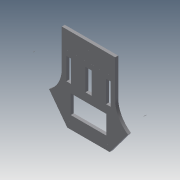
# Autodesk Inventor part: zak.-deska_ruka_(sablona)
Saved by Autodesk Inventor 2013 (Build 170138000, 138)
## iProperties
Created: 2013-02-01
Part Number: zak.-deska_ruka_(sablona)
Material: Generic
Document SubType Name: Modeling
Designer: idle-rug
Density: 1 g/cm^3
Author: idle-rug
Autodesk Inventor part; units mm, degrees
(part 1 of 2)
ref_plane "YZ Plane" through (0, 0, 0) normal (1, 0, 0) x (0, 1, 0)
ref_plane "XZ Plane" through (0, 0, 0) normal (0, 1, 0) x (-1, 0, 0)
ref_plane "XY Plane" through (0, 0, 0) normal (0, 0, 1) x (1, 0, 0)
sketch "Sketch1" plane through (0, 0, 0) normal (0, 1, 0) x (-1, 0, 0)
  line L0 (0, -20) -> (10, -20)
  line L1 (10, -20) -> (25, 0)
  line L2 (0, -20) -> (-10, -20)
  line L3 (-10, -20) -> (-25, 0)
  line L4 (25, 0) -> (25, 10)
  line L5 (0, 20) -> (15, 20)
  line L6 (15, 20) -> (25, 10)
  line L7 (0, 20) -> (-15, 20)
  line L8 (-25, 0) -> (-25, 10)
  line L9 (-25, 10) -> (-15, 20)
  line L10 (0, 20) -> (0, -20)
  point P0 (0, 0)
  dimension "d2" = 10
  dimension "d3" = 10
  dimension "d4" = 10
  dimension "d7" = 10
  constraints: 22 end point, 1 parallel
  measures "d2" distance of L0.start L0.end
  measures "d3" distance of L0.start L2.end
  measures "d4" distance of L1.end L4.end
  measures "d7" distance of L3.end L8.end
extrude "Extrusion1" add sketch "Sketch1" along normal blind 2
sketch "Sketch2" plane through (0, 2, 0) normal (0, 1, 0) x (1, 0, 0)
  circle A0 centre (-10, 10) radius 1.5
  circle A1 centre (10, 10) radius 1.5
  circle A2 centre (-16, 2) radius 1.5
  circle A3 centre (16, 2) radius 1.5
  point P0 (0, 0)
  dimension "d11" = 3
  dimension "d12" = 3
  dimension "d14" = 3
  dimension "d15" = 3
  constraints: 4 centre point
  measures "d11" diameter of A0
  measures "d12" diameter of A1
  measures "d14" diameter of A2
  measures "d15" diameter of A3
extrude "Extrusion2" cut sketch "Sketch2" against normal blind 10
sketch "Sketch4" plane through (0, 2, 0) normal (0, 1, 0) x (1, 0, 0)
  line L0 (25, -10) -> (25, 0) projected
  line L1 (-10, 20) -> (-10, 14)
  circle A0 centre (-10, 14) radius 1.5
  line L2 (10, 20) -> (10, 14)
  circle A1 centre (10, 14) radius 1.5
  point P0 (0, 0)
  dimension "d20" = 6
  dimension "d21" = 3
  dimension "d22" = 6
  dimension "d23" = 3
  constraints: 4 end point, 2 centre point, 2 coincident, 2 parallel
  measures "d20" distance of L1.start L1.end
  measures "d21" diameter of A0
  measures "d22" distance of L2.start L2.end
  measures "d23" diameter of A1
extrude "Extrusion3" cut sketch "Sketch4" against normal blind 10
sketch "Sketch5" plane through (0, 2, 0) normal (0, 1, 0) x (1, 0, 0)
  circle A0 centre (-10, 10) radius 1.5 projected
  circle A1 centre (10, 10) radius 1.5 projected
extrude "Extrusion4" add sketch "Sketch5" against normal blind 2
sketch "Sketch6" plane through (0, 2, 0) normal (0, 1, 0) x (1, 0, 0)
  circle A0 centre (-19, 2) radius 1.5
  circle A1 centre (19, 2) radius 1.5
  dimension "d34" = 3
  dimension "d36" = 3
  constraints: 2 centre point
  measures "d34" diameter of A0
  measures "d36" diameter of A1
extrude "Extrusion5" cut sketch "Sketch6" against normal blind 2
sketch "Sketch7" plane through (0, 2, 0) normal (0, 1, 0) x (1, 0, 0)
  circle A0 centre (-16, 2) radius 1.5 projected
  circle A1 centre (16, 2) radius 1.5 projected
  point P0 (-17.5, 2)
  point P1 (17.5, 2)
  point P2 (0, 0)
  constraints: 2 horizontal alignment
extrude "Extrusion6" add sketch "Sketch7" against normal blind 2
sketch "Sketch9" plane through (0, 2, 0) normal (0, 1, 0) x (1, 0, 0)
  line L0 (0, -2) -> (0, -4)
  circle A0 centre (0, -4) radius 2
  line L1 (-2, -4) -> (-2, -16)
  line L2 (-2, -16) -> (2, -16)
  line L3 (2, -4) -> (2, -16)
  circle A1 centre (0, -16) radius 2
  point P0 (0, 0)
  dimension "d48" = 2
  dimension "d49" = 4
  dimension "d51" = 12
  dimension "d52" = 4
  constraints: 8 end point, 2 centre point, 2 point on circle, 1 coincident, 1 midpoint, 1 perpendicular, 1 tangent
  measures "d48" distance of L0.start L0.end
  measures "d49" diameter of A0
  measures "d51" distance of L1.start L1.end
  measures "d52" diameter of A1
extrude "Extrusion7" cut sketch "Sketch9" against normal blind 2
sketch "Sketch10" plane through (0, 2, 0) normal (0, 1, 0) x (1, 0, 0)
  line L0 (-2, -16) -> (-2, -4) projected
  arc A0 (2, -4) -> (-2, -4) centre (0, -4) ccw projected
  line L1 (2, -4) -> (2, -16) projected
  arc A1 (-2, -16) -> (2, -16) centre (0, -16) ccw projected
  line L2 (25, -10) -> (25, 0) projected
  line L3 (0, -2) -> (0, -3.8)
  line L4 (0, -3.8) -> (0, -5.8)
  circle A2 centre (0, -5.8) radius 2
  point P0 (0, 0)
  dimension "d55" = 1.8
  dimension "d56" = 2
  dimension "d57" = 4
  constraints: 4 end point, 1 centre point, 1 coincident, 1 parallel, 1 point on circle, 1 point on line
  measures "d55" distance of L3.start L3.end
  measures "d56" distance of L3.end L4.end
  measures "d57" diameter of A2
extrude "Extrusion8" add sketch "Sketch10" against normal blind 2 contours L0 A2 L1 A1 | L0 A0 L3 A2 | L3 A0 L1 A2
sketch "Sketch11" plane through (0, 2, 0) normal (0, 1, 0) x (1, 0, 0)
  circle A0 centre (0, -5.8) radius 2 projected
  line L0 (25, -10) -> (25, 0) projected
  line L1 (2, -5.8) -> (2, -17.8)
  line L2 (2, -17.8) -> (-2, -17.8)
  line L3 (-2, -17.8) -> (-2, -5.8)
  circle A1 centre (0, -17.8) radius 2
  point P0 (0, 0)
  dimension "d60" = 12
  dimension "d61" = 4
  dimension "d62" = 4
  constraints: 6 end point, 2 point on circle, 2 tangent, 1 centre point, 1 midpoint, 1 parallel, 1 perpendicular
  measures "d60" distance of L1.start L1.end
  measures "d61" distance of L1.end L2.end
  measures "d62" diameter of A1
extrude "Extrusion9" cut sketch "Sketch11" against normal blind 2
sketch "Sketch12" plane through (0, 2, 0) normal (0, 1, 0) x (1, 0, 0)
  line L0 (-2, -17.8) -> (-2, -5.8) projected
  arc A0 (2, -5.8) -> (-2, -5.8) centre (0, -5.8) ccw projected
  line L1 (2, -5.8) -> (2, -17.8) projected
  arc A1 (-2, -17.8) -> (2, -17.8) centre (0, -17.8) ccw projected
  line L2 (-2, -5.8) -> (-2, -16.2)
  line L3 (-2, -16.2) -> (2, -16.2)
  line L4 (2, -16.2) -> (2, -5.8)
  line L5 (-2, -5.8) -> (2, -5.8)
  point P0 (0, 0)
  dimension "d65" = 16
  dimension "d66" = 12
  dimension "d67" = 10.4
  constraints: 8 end point, 2 perpendicular, 2 point on line, 1 collinear, 1 tangent
  measures "d66" distance of A1.centre A0.centre
  measures "d67" distance of L0.end L2.end
extrude "Extrusion10" add sketch "Sketch12" against normal blind 2 contours L0 L3 L1 A1
sketch "Sketch13" plane through (0, 2, 0) normal (0, 1, 0) x (1, 0, 0)
  line L0 (2, -16.2) -> (-2, -16.2) projected
  circle A0 centre (0, -16.2) radius 2
  point P0 (0, 0)
  dimension "d70" = 4
  constraints: 1 centre point, 1 midpoint
  measures "d70" diameter of A0
extrude "Extrusion11" cut sketch "Sketch13" against normal blind 2
sketch "Sketch14" plane through (0, 0, 0) normal (0, -1, 0) x (1, 0, 0)
  line L0 (15, 20) -> (25, 10) projected
  line L1 (-15, 20) -> (15, 20) projected
  line L2 (-25, 10) -> (-15, 20) projected
  line L3 (-25, 0) -> (-25, 10) projected
  line L4 (-15, 20) -> (-15, 40)
  line L5 (-15, 40) -> (15, 40)
  line L6 (15, 40) -> (15, 20)
  line L7 (15, 40) -> (25, 10)
  line L8 (-25, 10) -> (-15, 40)
  point P0 (0, 0)
  dimension "d74" = 20
  dimension "d75" = 30
  constraints: 10 end point, 1 parallel, 1 perpendicular
  measures "d74" distance of L1.start L4.end
  measures "d75" distance of L4.end L5.end
extrude "Extrusion12" add sketch "Sketch14" against normal blind 2
sketch "Sketch15" plane through (0, 2, 0) normal (0, 1, 0) x (1, 0, 0)
  circle A0 centre (-13.95, -27.8) radius 1.15
  circle A1 centre (13.95, -27.8) radius 1.15
  point P0 (0, 0)
  dimension "d83" = 2.3
  dimension "d84" = 2.3
  constraints: 2 centre point
  measures "d83" diameter of A0
  measures "d84" diameter of A1
extrude "Extrusion13" cut sketch "Sketch15" against normal blind 2
sketch "Sketch17" plane through (0, 0, 0) normal (0, -1, 0) x (1, 0, 0)
  line L0 (25, 10) -> (25, 0) projected
  line L1 (-25, 0) -> (-25, 10) projected
  arc A0 (-23.2, -2.4) -> (-19.7434, 25.7698) centre (-40.683, 14.0422) ccw
  arc A1 (19.7434, 25.7698) -> (23.2, -2.4) centre (40.683, 14.0422) ccw
  line L2 (-25, 0) -> (-23.2, -2.4)
  line L3 (19.7434, 25.7698) -> (25, 10)
  line L4 (25, 10) -> (25, 0)
  line L5 (23.2, -2.4) -> (25, 0)
  line L6 (-19.7434, 25.7698) -> (-25, 10)
  line L7 (-25, 0) -> (-25, 10)
  dimension "d90" = 24
  dimension "d92" = 24
  constraints: 12 end point, 4 point on circle, 2 centre point, 2 collinear
  measures "d90" radius of A0
  measures "d92" radius of A1
extrude "Extrusion14" cut sketch "Sketch17" against normal blind 2
sketch "Sketch18" plane through (0, 0, 0) normal (0, -1, 0) x (1, 0, 0)
  circle A0 centre (-11.2167, 36) radius 1.5
  circle A1 centre (11.2167, 36) radius 1.5
  circle A2 centre (0, -6.2) radius 1.5
  point P0 (0, 0)
  dimension "d97" = 3
  dimension "d98" = 3
  dimension "d100" = 3
  constraints: 3 centre point
  measures "d97" diameter of A0
  measures "d98" diameter of A1
  measures "d100" diameter of A2
extrude "Extrusion15" cut sketch "Sketch18" against normal blind 2
sketch "Sketch19" plane through (0, 0, 0) normal (0, -1, 0) x (1, 0, 0)
  circle A0 centre (11.2167, 36) radius 1.5 projected
  circle A1 centre (-11.2167, 36) radius 1.5 projected
  point P0 (0, 0)
extrude "Extrusion16" add sketch "Sketch19" against normal blind 2
sketch "Sketch20" plane through (0, 0, 0) normal (0, -1, 0) x (1, 0, 0)
  line L0 (19.7434, 25.7698) -> (15, 40) projected
  line L1 (-15, 40) -> (-19.7434, 25.7698) projected
  line L2 (10, -20) -> (-10, -20) projected
  line L3 (-19.7434, 25.7698) -> (-19.7434, 40)
  line L4 (-19.7434, 40) -> (19.7434, 40)
  line L5 (19.7434, 40) -> (19.7434, 25.7698)
  line L6 (-15, 40) -> (-19.7434, 25.7698)
  line L7 (19.7434, 25.7698) -> (15, 40)
  line L8 (-19.7434, 40) -> (-15, 40)
  line L9 (15, 40) -> (19.7434, 40)
  point P0 (0, 0)
  constraints: 14 end point, 3 collinear, 3 perpendicular
extrude "Extrusion17" add sketch "Sketch20" against normal blind 2
sketch "Sketch22" plane through (0, 0, 0) normal (0, -1, 0) x (1, 0, 0)
  circle A0 centre (0, -6.2) radius 1.5 projected
  circle A1 centre (19, -2) radius 1.5 projected
  circle A2 centre (-19, -2) radius 1.5 projected
  circle A3 centre (10, -14) radius 1.5 projected
  circle A4 centre (-10, -14) radius 1.5 projected
  circle A5 centre (13.95, 27.8) radius 1.15 projected
  circle A6 centre (-13.95, 27.8) radius 1.15 projected
  line L0 (19.7434, 25.7698) -> (19.7434, 40) projected
  line L1 (19.7434, 40) -> (-19.7434, 40) projected
  line L2 (-19.7434, 40) -> (-15.7434, 40)
  line L3 (-15.7434, 40) -> (-15.7434, 36)
  circle A7 centre (-15.7434, 36) radius 1.5
  circle A8 centre (-13.95, 27.8) radius 1.5
  circle A9 centre (-19, -2) radius 1.5
  circle A10 centre (0, -6.2) radius 1.5
  circle A11 centre (19, -2) radius 1.5
  circle A12 centre (-10, -14) radius 1.5
  circle A13 centre (10, -14) radius 1.5
  line L4 (19.7434, 36) -> (15.7434, 36)
  circle A14 centre (15.7434, 36) radius 1.5
  circle A15 centre (13.95, 27.8) radius 1.5
  circle A16 centre (15.7434, 36) radius 1.5
  point P0 (0, 0)
  dimension "d111" = 4
  dimension "d112" = 4
  dimension "d113" = 3
  dimension "d114" = 3
  dimension "d116" = 3
  dimension "d117" = 3
  dimension "d118" = 3
  dimension "d119" = 3
  dimension "d120" = 3
  dimension "d121" = 4
  dimension "d122" = 3
  dimension "d123" = 3
  dimension "d124" = 3
  constraints: 10 centre point, 10 coincident, 6 end point, 2 perpendicular, 2 point on line
  measures "d111" distance of L1.end L2.end
  measures "d112" distance of L2.end L3.end
  measures "d113" diameter of A7
  measures "d114" diameter of A8
  measures "d116" diameter of A9
  measures "d117" diameter of A10
  measures "d118" diameter of A11
  measures "d119" diameter of A12
  measures "d120" diameter of A13
  measures "d121" distance of L4.start L4.end
  measures "d122" diameter of A14
  measures "d123" diameter of A15
  measures "d124" diameter of A16
extrude "Extrusion18" cut sketch "Sketch22" against normal blind 2 contours A7 | A8 | A14 | A15
sketch "Sketch23" plane through (0, 0, 0) normal (0, -1, 0) x (1, 0, 0)
  circle A0 centre (-13.95, 27.8) radius 1.5 projected
  circle A1 centre (13.95, 27.8) radius 1.5 projected
  circle A2 centre (-13.95, 27.8) radius 1.15
  circle A3 centre (13.95, 27.8) radius 1.15
  circle A4 centre (10, 16.2) radius 2
  circle A5 centre (10, 5.8) radius 2
  line L0 (8, 16.2) -> (8, 5.8)
  line L1 (12, 16.2) -> (12, 5.8)
  line L2 (8, 5.8) -> (12, 5.8)
  line L3 (8, 16.2) -> (12, 16.2)
  point P0 (0, 0)
  dimension "d131" = 4
  dimension "d127" = 2.3
  dimension "d128" = 2.3
  dimension "d132" = 4
  constraints: 8 end point, 4 point on circle, 3 centre point, 2 coincident, 2 parallel, 2 vertical, 1 horizontal alignment, 1 perpendicular, 2 other
  measures "d127" diameter of A2
  measures "d128" diameter of A3
  measures "d132" diameter of A5
extrude "Extrusion19" cut sketch "Sketch23" against normal blind 2
sketch "Sketch24" plane through (0, 0, 0) normal (0, -1, 0) x (1, 0, 0)
  circle A0 centre (-13.95, 27.8) radius 1.5 projected
  circle A1 centre (13.95, 27.8) radius 1.5 projected
  circle A2 centre (-13.95, 27.8) radius 1.15
  circle A3 centre (13.95, 27.8) radius 1.15
  point P0 (0, 0)
  dimension "d135" = 2.3
  dimension "d136" = 2.3
  constraints: 2 centre point, 2 coincident
  measures "d135" diameter of A2
  measures "d136" diameter of A3
extrude "Extrusion20" add sketch "Sketch24" against normal blind 2
sketch "Sketch25" plane through (0, 0, 0) normal (0, -1, 0) x (1, 0, 0)
  circle A0 centre (0, -14) radius 1.5
  point P0 (0, 0)
  dimension "d139" = 3
  constraints: 1 centre point
  measures "d139" diameter of A0
extrude "Extrusion21" cut sketch "Sketch25" against normal blind 2
sketch "Sketch26" plane through (0, 0, 0) normal (0, -1, 0) x (1, 0, 0)
  circle A0 centre (0, -6.2) radius 1.5 projected
  point P0 (0, 0)
extrude "Extrusion22" add sketch "Sketch26" against normal blind 2
sketch "Sketch27" plane through (0, 0, 0) normal (0, -1, 0) x (1, 0, 0)
  arc A0 (19.7434, 25.7698) -> (23.2, -2.4) centre (40.683, 14.0422) ccw projected
  line L0 (19.7434, 25.7698) -> (19.7434, 40) projected
  line L1 (-19.7434, 40) -> (-19.7434, 25.7698) projected
  arc A1 (-23.2, -2.4) -> (-19.7434, 25.7698) centre (-40.683, 14.0422) ccw projected
  line L2 (0, 40) -> (-20, 40)
  line L3 (-20, 40) -> (-20, 26)
  line L4 (0, 40) -> (20, 40)
  line L5 (20, 40) -> (20, 26)
  arc A2 (-23.2, -2.4) -> (-20, 26) centre (-40.7609, 13.959) ccw
  arc A3 (20, 26) -> (23.2, -2.4) centre (40.7609, 13.959) ccw
  arc A4 (-23.2, -2.4) -> (-19.7434, 25.7698) centre (-40.683, 14.0422) ccw
  line L6 (-19.7434, 40) -> (-19.7434, 25.7698)
  line L7 (-20, 40) -> (-19.7434, 40)
  line L8 (19.7434, 40) -> (20, 40)
  line L9 (20, 40) -> (20, 26)
  line L10 (19.7434, 40) -> (19.7434, 25.7698)
  arc A5 (19.7434, 25.7698) -> (23.2, -2.4) centre (40.683, 14.0422) ccw
  point P0 (0, 0)
  dimension "d144" = 20
  dimension "d145" = 14
  dimension "d146" = 20
  dimension "d147" = 24
  dimension "d148" = 24
  constraints: 18 end point, 8 point on circle, 4 centre point, 3 collinear, 3 concentric, 3 perpendicular
  measures "d144" distance of L2.start L2.end
  measures "d145" distance of L2.end L3.end
  measures "d146" distance of L2.start L4.end
  measures "d147" radius of A2
  measures "d148" radius of A3
extrude "Extrusion23" add sketch "Sketch27" against normal blind 2
sketch "Sketch28" plane through (0, 0, 0) normal (0, -1, 0) x (1, 0, 0)
  circle A0 centre (15.7434, 36) radius 1.5 projected
  circle A1 centre (-15.7434, 36) radius 1.5 projected
  point P0 (0, 0)
extrude "Extrusion24" add sketch "Sketch28" against normal blind 2
sketch "Sketch29" plane through (0, 0, 0) normal (0, -1, 0) x (1, 0, 0)
  line L0 (20, 40) -> (16, 40)
  line L1 (20, 36) -> (20, 40)
  line L2 (-20, 40) -> (-16, 40)
  line L3 (-20, 36) -> (-20, 40)
  circle A0 centre (-16, 36) radius 1.5
  circle A1 centre (16, 36) radius 1.5
  point P0 (0, 0)
  dimension "d157" = 3
  dimension "d158" = 3
  constraints: 8 end point, 2 centre point, 2 horizontal
  measures "d157" diameter of A0
  measures "d158" diameter of A1
extrude "Extrusion25" cut sketch "Sketch29" against normal blind 2
sketch "Sketch30" plane through (0, 0, 0) normal (0, -1, 0) x (1, 0, 0)
  arc A0 (20, 26) -> (23.2, -2.4) centre (40.7609, 13.959) ccw projected
  arc A1 (-23.2, -2.4) -> (-20, 26) centre (-40.7609, 13.959) ccw projected
  arc A2 (20, 26) -> (23.2, -2.4) centre (35.5049, 13.3667) ccw
  arc A3 (-23.2, -2.4) -> (-20, 26) centre (-35.5049, 13.3667) ccw
  arc A4 (-23.2, -2.4) -> (-20, 26) centre (-40.7609, 13.959) ccw
  arc A5 (20, 26) -> (23.2, -2.4) centre (40.7609, 13.959) ccw
  point P0 (0, 0)
  dimension "d161" = 20
  dimension "d162" = 20
  constraints: 9 point on circle, 4 centre point, 2 concentric
  measures "d161" radius of A2
  measures "d162" radius of A3
extrude "Extrusion26" cut sketch "Sketch30" against normal blind 2
sketch "Sketch31" plane through (0, 0, 0) normal (0, -1, 0) x (1, 0, 0)
  circle A0 centre (-16, 36) radius 1.5 projected
  circle A1 centre (16, 36) radius 1.5 projected
  point P0 (0, 0)
extrude "Extrusion27" add sketch "Sketch31" against normal blind 2
sketch "Sketch32" plane through (0, 0, 0) normal (0, -1, 0) x (1, 0, 0)
  line L0 (-20, 40) -> (-17, 40)
  line L1 (-17, 40) -> (-17, 37)
  line L2 (-17, 37) -> (-20, 37)
  line L3 (-20, 37) -> (-20, 40)
  line L4 (20, 40) -> (17, 40)
  line L5 (17, 40) -> (17, 37)
  line L6 (17, 37) -> (20, 37)
  line L7 (20, 37) -> (20, 40)
  circle A0 centre (17, 37) radius 1.25
  circle A1 centre (-17, 37) radius 1.25
  point P0 (0, 0)
  dimension "d167" = 3
  dimension "d168" = 3
  dimension "d169" = 3
  dimension "d170" = 3
  dimension "d171" = 2.5
  dimension "d172" = 2.5
  constraints: 16 end point, 4 parallel, 2 centre point, 2 coincident, 2 horizontal, 2 perpendicular
  measures "d167" distance of L1.end L2.end
  measures "d168" distance of L0.end L1.end
  measures "d169" distance of L6.end L5.end
  measures "d170" distance of L5.end L4.end
  measures "d171" diameter of A0
  measures "d172" diameter of A1
extrude "Extrusion28" cut sketch "Sketch32" against normal blind 2 contours A1 L2 L1 | L1 L2 A1 | A0 L6 L5 | L5 L6 A0
sketch "Sketch33" plane through (-20, 0, 40) normal (0, 0, 1) x (1, 0, 0)
  line L0 (40, 0) -> (0, 0) projected
  line L1 (40, 0) -> (40, 2) projected
  line L2 (0, 2) -> (40, 2) projected
  line L3 (0, 0) -> (0, 2) projected
  point P0 (20, 0)
extrude "Extrusion29" add sketch "Sketch33" along normal blind 2
sketch "Sketch34" plane through (0, 2, 0) normal (0, 1, 0) x (1, 0, 0)
  arc A0 (23.2, 2.4) -> (20, -26) centre (35.5049, -13.3667) ccw projected
  line L0 (23.2, 2.4) -> (10, 20) projected
  line L1 (10, 20) -> (-10, 20) projected
  line L2 (-10, 20) -> (-23.2, 2.4) projected
  arc A1 (-20, -26) -> (-23.2, 2.4) centre (-35.5049, -13.3667) ccw projected
  line L3 (-20, -26) -> (-20, -42) projected
  line L4 (20, -42) -> (-20, -42) projected
  line L5 (20, -26) -> (20, -42) projected
  line L6 (0, 20) -> (-12.5, 20)
  line L7 (0, 20) -> (12.5, 20)
  line L8 (20, -42) -> (22.5, -42)
  line L9 (-20, -42) -> (-22.5, -42)
  line L10 (-22.5, -42) -> (-22.5, -26)
  line L11 (22.5, -42) -> (22.5, -26)
  line L12 (-12.5, 20) -> (-24.5, 4)
  line L13 (12.5, 20) -> (24.5, 4)
  arc A2 (-22.5, -26) -> (-24.5, 4) centre (-43.4307, -12.3287) ccw
  arc A3 (24.5, 4) -> (22.5, -26) centre (43.4307, -12.3287) ccw
  line L14 (20, -42) -> (20, -26)
  line L15 (-10, 20) -> (-23.2, 2.4)
  line L16 (10, 20) -> (23.2, 2.4)
  arc A4 (23.2, 2.4) -> (20, -26) centre (35.5049, -13.3667) ccw
  arc A5 (-20, -26) -> (-23.2, 2.4) centre (-35.5049, -13.3667) ccw
  line L17 (-20, -42) -> (-20, -26)
  point P0 (0, 0)
  dimension "d178" = 12.5
  dimension "d179" = 12.5
  dimension "d180" = 2.5
  dimension "d181" = 2.5
  dimension "d183" = 20
  dimension "d185" = 20
  dimension "d186" = 25
  dimension "d187" = 25
  constraints: 24 end point, 9 point on circle, 5 collinear, 4 centre point, 4 parallel, 2 concentric, 2 point on line, 1 midpoint, 1 perpendicular
  measures "d178" distance of L6.start L6.end
  measures "d179" distance of L6.start L7.end
  measures "d180" distance of L4.start L8.end
  measures "d181" distance of L3.end L9.end
  measures "d183" distance of L6.end L12.end
  measures "d185" distance of L7.end L13.end
  measures "d186" radius of A2
  measures "d187" radius of A3
extrude "Extrusion30" add sketch "Sketch34" against normal blind 2 contours L0 L7 L13 A3 L11 L8 L5 A0 | L9 L10 A2 L12 L6 L2 A1 L3
sketch "Sketch35" plane through (0, 2, 0) normal (0, 1, 0) x (1, 0, 0)
  line L0 (-12.5, 20) -> (-24.5, 4) projected
  arc A0 (-22.5, -26) -> (-24.5, 4) centre (-43.4307, -12.3287) ccw projected
  line L1 (22.5, -42) -> (22.5, -26) projected
  arc A1 (24.5, 4) -> (22.5, -26) centre (43.4307, -12.3287) ccw projected
  line L2 (24.5, 4) -> (12.5, 20) projected
  line L3 (-22.5, -42) -> (-24, -42)
  line L4 (-24, -42) -> (-24, -26)
  line L5 (22.5, -42) -> (24, -42)
  line L6 (24, -42) -> (24, -26)
  line L7 (12.5, 20) -> (14, 20)
  line L8 (14, 20) -> (26, 4)
  line L9 (-12.5, 20) -> (-14, 20)
  line L10 (-14, 20) -> (-26, 4)
  arc A2 (-24, -26) -> (-26, 4) centre (-43.6669, -12.2445) ccw
  arc A3 (26, 4) -> (24, -26) centre (43.6669, -12.2445) ccw
  line L11 (22.5, -42) -> (22.5, -26)
  line L12 (-22.5, -42) -> (-22.5, -26)
  line L13 (-24.5, 4) -> (-12.8, 19.6)
  line L14 (12.5, 20) -> (24.5, 4)
  arc A4 (-22.5, -26) -> (-24.5, 4) centre (-43.4307, -12.3287) ccw
  arc A5 (24.5, 4) -> (22.5, -26) centre (43.4307, -12.3287) ccw
  point P0 (0, 0)
  dimension "d190" = 1.5
  dimension "d191" = 1.5
  dimension "d192" = 1.5
  dimension "d193" = 20
  dimension "d194" = 1.5
  dimension "d195" = 20
  dimension "d196" = 24
  dimension "d197" = 24
  constraints: 24 end point, 8 point on circle, 7 equal length, 4 centre point, 4 perpendicular, 3 concentric, 1 point on line
  measures "d190" distance of L3.start L3.end
  measures "d191" distance of L1.start L5.end
  measures "d192" distance of L2.end L7.end
  measures "d193" distance of L7.end L8.end
  measures "d194" distance of L0.start L9.end
  measures "d195" distance of L9.end L10.end
  measures "d196" radius of A2
  measures "d197" radius of A3
extrude "Extrusion31" add sketch "Sketch35" against normal blind 2
sketch "Sketch36" plane through (0, 2, 0) normal (0, 1, 0) x (1, 0, 0)
  circle A0 centre (19, 2) radius 1.5 projected
  circle A1 centre (-19, 2) radius 1.5 projected
  circle A2 centre (10, 14) radius 1.5 projected
  circle A3 centre (-10, 14) radius 1.5 projected
  line L0 (-14, 20) -> (-26, 4) projected
  line L1 (26, 4) -> (14, 20) projected
  line L2 (10, 14) -> (19, 2)
  line L3 (-19, 2) -> (-10, 14)
  line L4 (-10, 14) -> (-12.72, 16.04)
  line L5 (-19, 2) -> (-21.72, 4.04)
  line L6 (10, 14) -> (12.72, 16.04)
  line L7 (12.72, 16.04) -> (21.72, 4.04)
  circle A4 centre (-21.72, 4.04) radius 1.5
  circle A5 centre (-12.72, 16.04) radius 1.5
  circle A6 centre (12.72, 16.04) radius 1.5
  circle A7 centre (21.72, 4.04) radius 1.5
  point P0 (0, 0)
  dimension "d200" = 3.4
  dimension "d201" = 3.4
  dimension "d202" = 3
  dimension "d203" = 3
  dimension "d204" = 3
  dimension "d205" = 3
  constraints: 12 end point, 4 centre point, 4 coincident, 4 parallel, 2 perpendicular
  measures "d200" distance of L3.end L4.end
  measures "d201" distance of L2.start L6.end
  measures "d202" diameter of A4
  measures "d203" diameter of A5
  measures "d204" diameter of A6
  measures "d205" diameter of A7
extrude "Extrusion32" cut sketch "Sketch36" against normal blind 2 contours A6 L7 L6 | L6 L7 A6 | A4 | A5 | A7
sketch "Sketch37" plane through (0, 2, 0) normal (0, 1, 0) x (1, 0, 0)
  circle A0 centre (19, 2) radius 1.5 projected
  circle A1 centre (-19, 2) radius 1.5 projected
  circle A2 centre (10, 14) radius 1.5 projected
  circle A3 centre (-10, 14) radius 1.5 projected
  point P0 (0, 0)
extrude "Extrusion33" add sketch "Sketch37" against normal blind 2
sketch "Sketch38" plane through (0, 2, 0) normal (0, 1, 0) x (1, 0, 0)
  arc A0 (-2, -16.2) -> (2, -16.2) centre (0, -16.2) ccw projected
  line L0 (-2, -16.2) -> (-2, -5.8) projected
  arc A1 (2, -5.8) -> (-2, -5.8) centre (0, -5.8) ccw projected
  line L1 (2, -5.8) -> (2, -16.2) projected
  line L2 (8, -16.2) -> (8, -5.8) projected
  arc A2 (12, -5.8) -> (8, -5.8) centre (10, -5.8) ccw projected
  line L3 (12, -5.8) -> (12, -16.2) projected
  arc A3 (8, -16.2) -> (12, -16.2) centre (10, -16.2) ccw projected
  line L4 (14, 20) -> (-14, 20) projected
  line L5 (24, -42) -> (24, -26) projected
  line L6 (0, 20) -> (0, 3)
  line L7 (0, 3) -> (0, -11.4)
  point P0 (0, 0)
  dimension "d210" = 17
  dimension "d211" = 14.4
  constraints: 4 end point, 1 collinear, 1 midpoint, 1 parallel
  measures "d210" distance of L6.start L6.end
  measures "d211" distance of L6.end L7.end
extrude "Extrusion34" add sketch "Sketch38" against normal blind 2
sketch "Sketch39" plane through (0, 2, 0) normal (0, 1, 0) x (1, 0, 0)
  line L0 (14, 20) -> (-14, 20) projected
  line L1 (24, -42) -> (24, -26) projected
  line L2 (0, 20) -> (0, 0.5)
  line L3 (0, 0.5) -> (0, -13.9)
  line L4 (0, 0.5) -> (0, -1)
  line L5 (0, -13.9) -> (0, -12.4)
  circle A0 centre (0, -12.4) radius 1.5
  circle A1 centre (0, -1) radius 1.5
  line L6 (-1.5, -1) -> (-1.5, -12.4)
  line L7 (1.5, -1) -> (1.5, -12.4)
  point P0 (0, 0)
  dimension "d214" = 19.5
  dimension "d215" = 14.4
  dimension "d216" = 1.5
  dimension "d217" = 1.5
  dimension "d218" = 3
  dimension "d219" = 3
  constraints: 12 end point, 4 point on circle, 3 tangent, 2 centre point, 2 coincident, 2 parallel, 2 point on line, 1 collinear, 1 midpoint
  measures "d214" distance of L2.start L2.end
  measures "d215" distance of L2.end L3.end
  measures "d216" distance of L2.end L4.end
  measures "d217" distance of L3.end L5.end
  measures "d218" diameter of A0
  measures "d219" diameter of A1
extrude "Extrusion35" cut sketch "Sketch39" against normal blind 2
sketch "Sketch40" plane through (0, 2, 0) normal (0, 1, 0) x (1, 0, 0)
  line L0 (-1.5, -12.4) -> (-1.5, -1) projected
  arc A0 (1.5, -1) -> (-1.5, -1) centre (0, -1) ccw projected
  line L1 (1.5, -1) -> (1.5, -12.4) projected
  arc A1 (-1.5, -12.4) -> (1.5, -12.4) centre (0, -12.4) ccw projected
  point P0 (0, 0)
extrude "Extrusion36" add sketch "Sketch40" against normal blind 2
sketch "Sketch41" plane through (0, 2, 0) normal (0, 1, 0) x (1, 0, 0)
  line L0 (14, 20) -> (-14, 20) projected
  line L1 (24, -42) -> (24, -26) projected
  line L2 (0, 20) -> (0, 0.5)
  line L3 (0, 0.5) -> (0, -1)
  circle A0 centre (0, -1) radius 1.5
  line L4 (0, 0.5) -> (0, -13.9)
  line L5 (0, -13.9) -> (0, -12.4)
  circle A1 centre (0, -12.4) radius 1.5
  line L6 (1.5, -12.4) -> (1.5, -1)
  line L7 (-1.5, -1) -> (-1.5, -12.4)
  point P0 (0, 0)
  dimension "d224" = 19.5
  dimension "d225" = 1.5
  dimension "d226" = 3
  dimension "d227" = 14.4
  dimension "d228" = 1.5
  dimension "d229" = 3
  constraints: 12 end point, 4 point on circle, 3 tangent, 2 centre point, 2 coincident, 2 collinear, 2 parallel, 1 midpoint, 1 point on line
  measures "d224" distance of L2.start L2.end
  measures "d225" distance of L2.end L3.end
  measures "d226" diameter of A0
  measures "d227" distance of L2.end L4.end
  measures "d228" distance of L4.end L5.end
  measures "d229" diameter of A1
extrude "Extrusion37" cut sketch "Sketch41" against normal blind 2
sketch "Sketch42" plane through (0, 2, 0) normal (0, 1, 0) x (1, 0, 0)
  circle A0 centre (0, 14) radius 1.5 projected
  point P0 (0, 0)
sketch "Sketch43" plane through (0, 2, 0) normal (0, 1, 0) x (1, 0, 0)
  line L0 (14, 20) -> (-14, 20) projected
  line L1 (24, -42) -> (24, -26) projected
  line L2 (0, 20) -> (0, 5.5)
  line L3 (0, 5.5) -> (-13.95, 5.5)
  line L4 (0, 5.5) -> (13.95, 5.5)
  circle A0 centre (-13.95, 5.5) radius 1.5
  circle A1 centre (13.95, 5.5) radius 1.5
  point P0 (0, 0)
  dimension "d236" = 14.5
  dimension "d237" = 13.95
  dimension "d238" = 13.95
  dimension "d239" = 3
  dimension "d241" = 3
  constraints: 6 end point, 2 centre point, 2 coincident, 1 collinear, 1 midpoint, 1 parallel, 1 perpendicular
  measures "d236" distance of L2.start L2.end
  measures "d237" distance of L2.end L3.end
  measures "d238" distance of L2.end L4.end
  measures "d239" diameter of A0
  measures "d241" diameter of A1
extrude "Extrusion38" add sketch "Sketch42" against normal blind 2
extrude "Extrusion39" cut sketch "Sketch43" against normal blind 2
sketch "Sketch44" plane through (0, 2, 0) normal (0, 1, 0) x (1, 0, 0)
  line L0 (1.5, -1) -> (1.5, -12.4) projected
  arc A0 (-1.5, -12.4) -> (1.5, -12.4) centre (0, -12.4) ccw projected
  line L1 (-1.5, -12.4) -> (-1.5, -1) projected
  arc A1 (1.5, -1) -> (-1.5, -1) centre (0, -1) ccw projected
  point P0 (0, 0)
extrude "Extrusion40" add sketch "Sketch44" against normal blind 2
sketch "Sketch45" plane through (0, 2, 0) normal (0, 1, 0) x (1, 0, 0)
  line L0 (-24, -42) -> (24, -42) projected
  line L1 (24, -42) -> (24, -26) projected
  line L2 (0, -42) -> (0, -20.4)
  line L3 (0, -20.4) -> (0, -6)
  line L4 (0, -20.4) -> (0, -18.4)
  line L5 (0, -6) -> (0, -8)
  circle A0 centre (0, -18.4) radius 2
  circle A1 centre (0, -8) radius 2
  line L6 (-2, -18.4) -> (-2, -8)
  line L7 (2, -8) -> (2, -18.4)
  point P0 (0, 0)
  dimension "d248" = 14.4
  dimension "d249" = 21.6
  dimension "d250" = 2
  dimension "d251" = 2
  dimension "d252" = 4
  dimension "d253" = 4
  constraints: 12 end point, 4 point on circle, 2 centre point, 2 coincident, 2 parallel, 2 point on line, 2 tangent, 1 midpoint
  measures "d248" distance of L2.end L3.end
  measures "d249" distance of L2.start L2.end
  measures "d250" distance of L2.end L4.end
  measures "d251" distance of L3.end L5.end
  measures "d252" diameter of A0
  measures "d253" diameter of A1
extrude "Extrusion41" cut sketch "Sketch45" against normal blind 2
sketch "Sketch46" plane through (0, 2, 0) normal (0, 1, 0) x (1, 0, 0)
  arc A0 (-24, -26) -> (-26, 4) centre (-43.6669, -12.2445) ccw projected
  arc A1 (26, 4) -> (24, -26) centre (43.6669, -12.2445) ccw projected
  arc A2 (-24, -26) -> (-26, 4) centre (-36.5932, -11.7729) ccw
  arc A3 (26, 4) -> (24, -26) centre (36.5932, -11.7729) ccw
  arc A4 (26, 4) -> (24, -26) centre (43.6669, -12.2445) ccw
  arc A5 (-24, -26) -> (-26, 4) centre (-43.6669, -12.2445) ccw
  point P0 (0, 0)
  dimension "d256" = 19
  dimension "d259" = 19
  constraints: 8 point on circle, 4 centre point, 2 concentric
  measures "d256" radius of A2
  measures "d259" radius of A3
extrude "Extrusion42" cut sketch "Sketch46" against normal blind 2
sketch "Sketch47" plane through (0, 2, 0) normal (0, 1, 0) x (1, 0, 0)
  arc A0 (2, -8) -> (-2, -8) centre (0, -8) ccw projected
  line L0 (2, -8) -> (2, -18.4) projected
  line L1 (0, -8) -> (10, -8)
  circle A1 centre (10, -8) radius 2
  circle A2 centre (10, -18.4) radius 2
  line L2 (8, -8) -> (8, -18.4)
  line L3 (12, -8) -> (12, -18.4)
  point P0 (0, 0)
  dimension "d262" = 10
  dimension "d263" = 4
  dimension "d264" = 4
  constraints: 6 end point, 4 point on circle, 2 centre point, 2 tangent, 1 coincident, 1 parallel, 1 perpendicular, 1 point on line
  measures "d262" distance of L1.start L1.end
  measures "d263" diameter of A1
  measures "d264" diameter of A2
extrude "Extrusion43" cut sketch "Sketch47" against normal blind 2
sketch "Sketch48" plane through (0, 2, 0) normal (0, 1, 0) x (1, 0, 0)
  circle A0 centre (-13.95, -27.8) radius 1.15 projected
  circle A1 centre (13.95, -27.8) radius 1.15 projected
  point P0 (0, 0)
extrude "Extrusion44" add sketch "Sketch48" against normal blind 2
sketch "Sketch49" plane through (0, 2, 0) normal (0, 1, 0) x (1, 0, 0)
  line L0 (-24, -26) -> (-24, -42) projected
  line L1 (-24, -42) -> (24, -42) projected
  line L2 (24, -42) -> (24, -26) projected
  circle A0 centre (17, -37) radius 1.25 projected
  circle A1 centre (-17, -37) radius 1.25 projected
  line L3 (-24, -26) -> (24, -26)
  line L4 (24, -26) -> (24, -42)
  line L5 (-24, -42) -> (24, -42)
  line L6 (-24, -26) -> (-24, -42)
  point P0 (0, 0)
  constraints: 8 end point, 3 collinear
extrude "Extrusion45" cut sketch "Sketch49" against normal blind 2
sketch "Sketch50" plane through (0, 2, 0) normal (0, 1, 0) x (1, 0, 0)
  line L0 (-24, -26) -> (24, -26) projected
  arc A0 (26, 4) -> (24, -26) centre (36.5932, -11.7729) ccw projected
  arc A1 (-24, -26) -> (-26, 4) centre (-36.5932, -11.7729) ccw projected
  line L1 (-17.5932, -11.7729) -> (-17.5932, -26)
  line L2 (-17.5932, -26) -> (-24, -26)
  line L3 (17.5932, -11.7729) -> (17.5932, -26)
  line L4 (24, -26) -> (17.5932, -26)
  arc A2 (26, 4) -> (24, -26) centre (36.5932, -11.7729) ccw
  arc A3 (-24, -26) -> (-26, 4) centre (-36.5932, -11.7729) ccw
  point P0 (0, 0)
  constraints: 8 end point, 7 point on circle, 2 centre point, 2 collinear, 2 concentric, 2 perpendicular, 2 point on line, 1 tangent
extrude "Extrusion46" cut sketch "Sketch50" against normal blind 2
sketch "Sketch51" plane through (0, 2, 0) normal (0, 1, 0) x (1, 0, 0)
  line L0 (-17.5932, -11.7729) -> (-17.5932, -26) projected
  line L1 (-17.5932, -26) -> (17.5932, -26) projected
  line L2 (17.5932, -26) -> (17.5932, -11.7729) projected
  line L3 (-17.5932, -26) -> (-17.5932, -20.4)
  line L4 (-17.5932, -26) -> (17.5932, -26)
  line L5 (17.5932, -26) -> (17.5932, -22.4)
  line L6 (17.5932, -22.4) -> (-17.5932, -22.4)
  line L7 (17.5932, -22.4) -> (17.5932, -26)
  line L8 (-17.5932, -22.4) -> (-17.5932, -26)
  point P0 (0, 0)
  dimension "d273" = 3.6
  constraints: 12 end point, 3 collinear, 2 perpendicular, 2 point on line
  measures "d273" distance of L1.end L5.end
extrude "Extrusion47" cut sketch "Sketch51" against normal blind 2
sketch "Sketch52" plane through (0, 2, 0) normal (0, 1, 0) x (1, 0, 0)
  line L0 (-17.5932, -22.4) -> (17.5932, -22.4) projected
  line L1 (17.5932, -22.4) -> (17.5932, -11.7729) projected
  line L2 (-17.5932, -11.7729) -> (-17.5932, -22.4) projected
  line L3 (-17.5932, -22.4) -> (-17.5932, -20.9)
  line L4 (-17.5932, -20.9) -> (17.5932, -20.9)
  line L5 (17.5932, -22.4) -> (17.5932, -20.9)
  line L6 (17.5932, -22.4) -> (-17.5932, -22.4)
  point P0 (0, 0)
  dimension "d276" = 1.5
  constraints: 8 end point, 2 point on line, 1 collinear, 1 parallel, 1 perpendicular
  measures "d276" distance of L0.start L3.end
extrude "Extrusion48" add sketch "Sketch52" along normal blind 10
fillet "Fillet1" radius 2 1 edges at (0, 0, 22.4)
sketch "Sketch53" plane through (0, 2, 0) normal (0, 1, 0) x (1, 0, 0)
  line L0 (-17.5932, -20.9) -> (17.5932, -20.9) projected
  line L1 (17.5932, -20.9) -> (17.5932, -11.7729) projected
  arc A0 (26, 4) -> (17.5932, -11.7729) centre (36.5932, -11.7729) ccw projected
  line L2 (26, 4) -> (14, 20) projected
  line L3 (14, 20) -> (-14, 20) projected
  line L4 (-14, 20) -> (-26, 4) projected
  arc A1 (-17.5932, -11.7729) -> (-26, 4) centre (-36.5932, -11.7729) ccw projected
  line L5 (-17.5932, -11.7729) -> (-17.5932, -20.9) projected
  line L6 (-2, -18.4) -> (-2, -8) projected
  arc A2 (2, -8) -> (-2, -8) centre (0, -8) ccw projected
  line L7 (2, -8) -> (2, -18.4) projected
  arc A3 (-2, -18.4) -> (2, -18.4) centre (0, -18.4) ccw projected
  circle A4 centre (-13.95, 5.5) radius 1.5 projected
  circle A5 centre (13.95, 5.5) radius 1.5 projected
  circle A6 centre (12.72, 16.04) radius 1.5 projected
  circle A7 centre (21.72, 4.04) radius 1.5 projected
  circle A8 centre (-21.72, 4.04) radius 1.5 projected
  circle A9 centre (-12.72, 16.04) radius 1.5 projected
  line L8 (8, -18.4) -> (8, -8) projected
  arc A10 (12, -8) -> (8, -8) centre (10, -8) ccw projected
  line L9 (12, -8) -> (12, -18.4) projected
  arc A11 (8, -18.4) -> (12, -18.4) centre (10, -18.4) ccw projected
  line L10 (6.5, -16.4) -> (13.5, -16.4)
  line L11 (13.5, -16.4) -> (13.5, -20.4)
  line L12 (13.5, -20.4) -> (6.5, -20.4)
  line L13 (6.5, -20.4) -> (6.5, -16.4)
  line L14 (6.5, -16.4) -> (13.5, -20.4) construction
  line L15 (13.5, -16.4) -> (6.5, -20.4) construction
  line L16 (13.5, -6) -> (6.5, -6)
  line L17 (6.5, -6) -> (6.5, -10)
  line L18 (6.5, -10) -> (13.5, -10)
  line L19 (13.5, -10) -> (13.5, -6)
  line L20 (13.5, -6) -> (6.5, -10) construction
  line L21 (6.5, -6) -> (13.5, -10) construction
  line L22 (3.5, -6) -> (-3.5, -6)
  line L23 (-3.5, -6) -> (-3.5, -10)
  line L24 (-3.5, -10) -> (3.5, -10)
  line L25 (3.5, -10) -> (3.5, -6)
  line L26 (3.5, -6) -> (-3.5, -10) construction
  line L27 (-3.5, -6) -> (3.5, -10) construction
  line L28 (3.5, -16.4) -> (-3.5, -16.4)
  line L29 (-3.5, -16.4) -> (-3.5, -20.4)
  line L30 (-3.5, -20.4) -> (3.5, -20.4)
  line L31 (3.5, -20.4) -> (3.5, -16.4)
  line L32 (3.5, -16.4) -> (-3.5, -20.4) construction
  line L33 (-3.5, -16.4) -> (3.5, -20.4) construction
  line L34 (6.5, -10) -> (6.5, -16.4)
  line L35 (6.5, -16.4) -> (13.5, -16.4)
  line L36 (13.5, -16.4) -> (13.5, -10)
  line L37 (13.5, -10) -> (6.5, -10)
  line L38 (-3.5, -10) -> (-3.5, -16.4)
  line L39 (-3.5, -16.4) -> (3.5, -16.4)
  line L40 (3.5, -16.4) -> (3.5, -10)
  line L41 (-3.5, -10) -> (3.5, -10)
  point P0 (0, 0)
  dimension "d322" = 7
  dimension "d323" = 7
  dimension "d324" = 4
  dimension "d325" = 7
  dimension "d326" = 4
  dimension "d327" = 7
  dimension "d328" = 4
  constraints: 64 end point, 10 equal length, 8 midpoint, 4 horizontal, 4 perpendicular
  measures "d322" distance of L11.end L12.end
  measures "d323" distance of L18.end L17.end
  measures "d324" distance of L17.end L16.end
  measures "d325" distance of L24.end L23.end
  measures "d326" distance of L23.end L22.end
  measures "d327" distance of L30.end L29.end
  measures "d328" distance of L29.end L28.end
extrude "Extrusion49" cut sketch "Sketch53" against normal blind 0.5 contours L5 A1 L4 L3 L2 A0 L1 L0 | A3 L30 L29 L28 L6 | L28 L38 L24 L6 | A3 L7 L28 L31 L30 | L24 L23 L22 A2 L6 | L7 L24 L40 L28 | L7 A2 L22 L25 L24 | A11 L12 L13 L10 L8 | L10 L34 L18 L8 | A11 L9 L10 L11 L12 | L18 L17 L16 A10 L8 | L9 L18 L36 L10 | L9 A10 L16 L19 L18
fillet "Fillet2" radius 0.5 1 edges at (0, 1.5, 20.9)
sketch "Sketch54" plane through (0, 0, 0) normal (0, -1, 0) x (1, 0, 0)
  line L0 (-17.5932, 20.4) -> (0, 20.4) projected
  arc A0 (2, 18.4) -> (0, 20.4) centre (0, 18.4) ccw projected
  line L1 (2, 18.4) -> (2, 8) projected
  arc A1 (-2, 8) -> (2, 8) centre (0, 8) ccw projected
  line L2 (-2, 8) -> (-2, 18.4) projected
  arc A2 (0, 20.4) -> (-2, 18.4) centre (0, 18.4) ccw projected
  line L3 (2, 16.4) -> (-2, 16.4)
  line L4 (-2, 16.4) -> (-2, 20.4)
  line L5 (-2, 20.4) -> (2, 20.4)
  line L6 (2, 20.4) -> (2, 16.4)
  line L7 (2, 16.4) -> (-2, 20.4) construction
  line L8 (-2, 16.4) -> (2, 20.4) construction
  line L9 (2, 10) -> (-2, 10)
  line L10 (-2, 10) -> (-2, 6)
  line L11 (-2, 6) -> (2, 6)
  line L12 (2, 6) -> (2, 10)
  line L13 (2, 10) -> (-2, 6) construction
  line L14 (-2, 10) -> (2, 6) construction
  point P0 (0, 0)
  constraints: 24 end point, 4 midpoint, 4 parallel, 2 horizontal, 2 perpendicular, 2 point on line
extrude "Extrusion50" cut sketch "Sketch54" against normal blind 1.5 contours A0 L1 L3 L2 A2 | L3 L1 L9 L2 | L9 L1 A1 L2 | A1 L11 L10 | L12 L11 A1
sketch "Sketch55" plane through (0, 0, 0) normal (0, -1, 0) x (1, 0, 0)
  line L0 (-2, 6) -> (-2, 18.4) projected
  arc A0 (2, 18.4) -> (0, 20.4) centre (0, 18.4) ccw projected
  line L1 (2, 20.3989) -> (-2, 20.3989)
  line L2 (-2, 20.3989) -> (-2, 16.4011)
  line L3 (-2, 16.4011) -> (2, 16.4011)
  line L4 (2, 16.4011) -> (2, 20.3989)
  line L5 (2, 20.3989) -> (-2, 16.4011) construction
  line L6 (-2, 20.3989) -> (2, 16.4011) construction
  point P0 (0, 0)
  constraints: 12 end point, 2 midpoint, 2 parallel, 1 horizontal, 1 perpendicular, 1 point on line
extrude "Extrusion51" cut sketch "Sketch55" against normal blind 1.5
sketch "Sketch56" plane through (0, 0, 0) normal (0, -1, 0) x (1, 0, 0)
  line L0 (0.0665, 20.3989) -> (2, 20.3989) projected
  line L1 (2, 20.3989) -> (2, 6) projected
  line L2 (2, 6) -> (-2, 6) projected
  line L3 (-2, 6) -> (-2, 20.3989) projected
  line L4 (-2, 20.3989) -> (-0.0665, 20.3989) projected
  arc A0 (0, 20.4) -> (-0.0665, 20.3989) centre (0, 18.4) ccw projected
  arc A1 (0.0665, 20.3989) -> (0, 20.4) centre (0, 18.4) ccw projected
  line L5 (-2, 20.3989) -> (2, 20.3989)
  line L6 (2, 20.3989) -> (2, 4.3989)
  line L7 (2, 4.3989) -> (-2, 4.3989)
  line L8 (-2, 4.3989) -> (-2, 20.3989)
  point P0 (8, 8)
  point P1 (8, 18.4)
  point P2 (0, 0)
  dimension "d287" = 10.4
  dimension "d288" = 14.3989
  dimension "d289" = 16
  constraints: 8 end point, 2 parallel, 1 horizontal, 1 perpendicular, 1 point on line
  measures "d287" distance of point (8, 8) point (8, 18.4)
  measures "d288" distance of L2.end L3.end
  measures "d289" distance of L5.end L6.end
extrude "Extrusion52" cut sketch "Sketch56" against normal blind 1.5 contours L6 L7 L8 L2
sketch "Sketch57" plane through (0, 0, 0) normal (0, -1, 0) x (1, 0, 0)
  arc A0 (8, 8) -> (12, 8) centre (10, 8) ccw projected
  line L0 (8, 8) -> (8, 18.4) projected
  arc A1 (10, 20.4) -> (8, 18.4) centre (10, 18.4) ccw projected
  line L1 (12, 20.3388) -> (8, 20.3388)
  line L2 (8, 20.3388) -> (8, 16.4612)
  line L3 (8, 16.4612) -> (12, 16.4612)
  line L4 (12, 16.4612) -> (12, 20.3388)
  line L5 (12, 20.3388) -> (8, 16.4612) construction
  line L6 (8, 20.3388) -> (12, 16.4612) construction
  line L7 (12, 10) -> (8, 10)
  line L8 (8, 10) -> (8, 6)
  line L9 (8, 6) -> (12, 6)
  line L10 (12, 6) -> (12, 10)
  line L11 (12, 10) -> (8, 6) construction
  line L12 (8, 10) -> (12, 6) construction
  line L13 (12, 11.6011) -> (8, 11.6011)
  line L14 (8, 11.6011) -> (8, 4.3989)
  line L15 (8, 4.3989) -> (12, 4.3989)
  line L16 (12, 4.3989) -> (12, 11.6011)
  line L17 (12, 11.6011) -> (8, 4.3989) construction
  line L18 (8, 11.6011) -> (12, 4.3989) construction
  point P0 (0, 0)
  constraints: 36 end point, 6 midpoint, 6 parallel, 3 horizontal, 3 perpendicular, 2 point on line
extrude "Extrusion53" cut sketch "Sketch57" against normal blind 1.5
sketch "Sketch58" plane through (0, 12, 0) normal (0, 1, 0) x (1, 0, 0)
  line L0 (-17.5932, -22.4) -> (17.5932, -22.4) projected
  line L1 (17.5932, -22.4) -> (17.5932, -20.9) projected
  line L2 (17.5932, -20.9) -> (-17.5932, -20.9) projected
  line L3 (-17.5932, -20.9) -> (-17.5932, -22.4) projected
  point P0 (0, 0)
extrude "Extrusion54" cut sketch "Sketch58" against normal blind 10
sketch "Sketch59" plane through (0, 2, 0) normal (0, 1, 0) x (1, 0, 0)
  line L0 (17.5932, -22.4) -> (-17.5932, -22.4) projected
  line L1 (17.5932, -20.9) -> (17.5932, -22.4) projected
  line L2 (-17.5932, -20.9) -> (17.5932, -20.9) projected
  line L3 (-17.5932, -22.4) -> (-17.5932, -20.9) projected
  point P0 (0, 0)
extrude "Extrusion55" cut sketch "Sketch59" against normal blind 10
sketch "Sketch60" plane through (0, 1.5, 0) normal (0, 1, 0) x (1, 0, 0)
  line L0 (-17.5932, -20.4) -> (17.5932, -20.4)
  line L1 (17.5932, -20.4) -> (17.5932, -21.0619)
  line L2 (17.5932, -21.0619) -> (-17.5932, -21.0619)
  line L3 (-17.5932, -21.0619) -> (-17.5932, -20.4)
  point P0 (0, 0)
  constraints: 8 end point, 2 parallel, 1 horizontal, 1 perpendicular
extrude "Extrusion56" add sketch "Sketch60" along normal blind 10
sketch "Sketch61" plane through (0, 11.5, 0) normal (0, 1, 0) x (1, 0, 0)
  line L0 (-17.5932, -20.4) -> (-17.5932, -21.0619) projected
  line L1 (-17.5932, -21.0619) -> (17.5932, -21.0619) projected
  line L2 (17.5932, -21.0619) -> (17.5932, -20.4) projected
  line L3 (17.5932, -20.4) -> (-17.5932, -20.4) projected
  point P0 (0, 0)
extrude "Extrusion57" cut sketch "Sketch61" against normal blind 20
sketch "Sketch62" plane through (0, 1.5, 0) normal (0, 1, 0) x (1, 0, 0)
  line L0 (12, -4.3989) -> (12, -20.3388) projected
  line L1 (12, -20.3388) -> (10.4911, -20.3388) projected
  arc A0 (10, -20.4) -> (10.4911, -20.3388) centre (10, -18.4) ccw projected
  line L2 (17.5932, -20.4) -> (10, -20.4) projected
  line L3 (0, -20.4) -> (-17.5932, -20.4) projected
  arc A1 (-0.0665, -20.3989) -> (0, -20.4) centre (0, -18.4) ccw projected
  line L4 (-0.0665, -20.3989) -> (-2, -20.3989) projected
  line L5 (-2, -20.3989) -> (-2, -4.3989) projected
  line L6 (-2, -4.3989) -> (2, -4.3989) projected
  line L7 (2, -4.3989) -> (2, -20.3989) projected
  line L8 (2, -20.3989) -> (0.0665, -20.3989) projected
  arc A2 (0, -20.4) -> (0.0665, -20.3989) centre (0, -18.4) ccw projected
  line L9 (10, -20.4) -> (0, -20.4) projected
  arc A3 (9.5089, -20.3388) -> (10, -20.4) centre (10, -18.4) ccw projected
  line L10 (9.5089, -20.3388) -> (8, -20.3388) projected
  line L11 (8, -20.3388) -> (8, -4.3989) projected
  line L12 (8, -4.3989) -> (12, -4.3989) projected
  line L13 (3.5, -4.3989) -> (3.5, -20.4)
  line L14 (-3.5, -4.3989) -> (-3.5, -20.4)
  line L15 (-3.5, -20.4) -> (3.5, -20.4)
  line L16 (6.5, -4.3989) -> (6.5, -20.4)
  line L17 (13.5, -4.3989) -> (13.5, -20.4)
  line L18 (7.1277, -20.4) -> (13.5, -20.4)
  line L19 (-3.5, -4.3989) -> (3.5, -4.3989)
  line L20 (6.5, -4.3989) -> (13.5, -4.3989)
  line L21 (6.5, -20.4) -> (13.5, -20.4)
  point P0 (0, 0)
  constraints: 18 end point, 6 perpendicular, 5 point on line, 2 collinear, 1 parallel
extrude "Extrusion58" add sketch "Sketch62" against normal blind 1.5 contours L0 L1 A0 A3 L10 L11 L12 | L3 L5 L6 L7 L8 A2
sketch "Sketch63" plane through (0, 1.5, 0) normal (0, 1, 0) x (1, 0, 0)
  line L0 (13.5932, -20.4) -> (6.5932, -20.4)
  line L1 (6.5932, -20.4) -> (6.5932, -4.4)
  line L2 (6.5932, -4.4) -> (13.5932, -4.4)
  line L3 (13.5932, -4.4) -> (13.5932, -20.4)
  line L4 (3.5932, -20.4) -> (-3.4068, -20.4)
  line L5 (-3.4068, -20.4) -> (-3.4068, -4.4)
  line L6 (-3.4068, -4.4) -> (3.5932, -4.4)
  line L7 (3.5932, -4.4) -> (3.5932, -20.4)
  point P0 (17.5932, -20.4)
  point P1 (0, 0)
  dimension "d308" = 4
  dimension "d309" = 7
  dimension "d310" = 16
  dimension "d311" = 3
  dimension "d312" = 7
  dimension "d313" = 16
  constraints: 16 end point, 4 parallel, 2 horizontal, 2 perpendicular
  measures "d308" distance of point (17.593, -20.4) L0.start
  measures "d309" distance of L1.end L2.end
  measures "d310" distance of L0.end L1.end
  measures "d311" distance of L0.end L4.start
  measures "d312" distance of L5.end L6.end
  measures "d313" distance of L4.end L5.end
extrude "Extrusion59" cut sketch "Sketch63" against normal blind 1.5
sketch "Sketch64" plane through (0, 1.5, 0) normal (0, 1, 0) x (1, 0, 0)
  line L0 (17.5932, -20.4) -> (13.5932, -20.4) projected
  line L1 (-17.5932, -20.4) -> (17.5932, -20.4)
  line L2 (17.5932, -20.4) -> (17.5932, -25.4)
  line L3 (17.5932, -25.4) -> (-17.5932, -25.4)
  line L4 (-17.5932, -25.4) -> (-17.5932, -20.4)
  point P0 (0, 0)
  dimension "d316" = 5
  constraints: 8 end point, 2 perpendicular, 1 collinear, 1 parallel
  measures "d316" distance of L0.start L2.end
extrude "Extrusion60" add sketch "Sketch64" against normal blind 1.5
sketch "Sketch65" plane through (0, 1.5, 0) normal (0, 1, 0) x (1, 0, 0)
  line L0 (17.5932, -25.4) -> (17.5932, -11.7729) projected
  line L1 (-17.5932, -25.4) -> (-17.5932, -11.7729) projected
  line L2 (-17.5932, -25.4) -> (17.5932, -25.4) projected
  line L3 (-17.5932, -25.4) -> (-17.5932, -23.9)
  line L4 (-17.5932, -23.9) -> (17.5932, -23.9)
  line L5 (17.5932, -25.4) -> (17.5932, -23.9)
  line L6 (17.5932, -25.4) -> (-17.5932, -25.4)
  point P0 (0, 0)
  dimension "d319" = 1.5
  constraints: 8 end point, 2 perpendicular, 2 point on line, 1 collinear
  measures "d319" distance of L1.start L3.end
extrude "Extrusion61" add sketch "Sketch65" along normal blind 10
sketch "Sketch66" plane through (0, 1.5, 0) normal (0, 1, 0) x (1, 0, 0)
  line L0 (3.5932, -20.4) -> (-3.4068, -20.4) projected
  line L1 (-3.4068, -20.4) -> (-3.4068, -4.4) projected
  line L2 (-3.4068, -4.4) -> (3.5932, -4.4) projected
  line L3 (3.5932, -4.4) -> (3.5932, -20.4) projected
  line L4 (13.5932, -20.4) -> (6.5932, -20.4) projected
  line L5 (6.5932, -20.4) -> (6.5932, -4.4) projected
  line L6 (6.5932, -4.4) -> (13.5932, -4.4) projected
  line L7 (13.5932, -4.4) -> (13.5932, -20.4) projected
  point P0 (0, 0)
extrude "Extrusion62" add sketch "Sketch66" against normal blind 1.5
sketch "Sketch68" plane through (0, 1.5, 0) normal (0, 1, 0) x (1, 0, 0)
  line L0 (17.5932, -23.9) -> (17.5932, -11.7729) projected
  line L1 (17.5932, -23.9) -> (17.5932, -19.9)
  line L2 (13.4642, -19.9) -> (6.4642, -19.9)
  line L3 (6.4642, -19.9) -> (6.4642, -4.9)
  line L4 (6.4642, -4.9) -> (13.4642, -4.9)
  line L5 (13.4642, -4.9) -> (13.4642, -19.9)
  line L6 (6.4642, -19.9) -> (3.3922, -19.9)
  line L7 (3.3922, -19.9) -> (-3.6078, -19.9)
  line L8 (-3.6078, -19.9) -> (-3.6078, -4.9)
  line L9 (-3.6078, -4.9) -> (3.3922, -4.9)
  line L10 (3.3922, -4.9) -> (3.3922, -19.9)
  point P0 (0, 0)
  dimension "d331" = 4
  dimension "d332" = 4.129
  dimension "d333" = 7
  dimension "d335" = 3.072
  dimension "d336" = 7
  dimension "d337" = 15
  constraints: 20 end point, 4 parallel, 3 perpendicular, 2 horizontal, 1 point on line
  measures "d331" distance of L0.start L1.end
  measures "d332" distance of L1.end L2.start
  measures "d333" distance of L3.end L4.end
  measures "d335" distance of L2.end L6.end
  measures "d336" distance of L8.end L9.end
  measures "d337" distance of L7.end L8.end
extrude "Extrusion63" cut sketch "Sketch68" against normal blind 1.5
sketch "Sketch69" plane through (0, 1.5, 0) normal (0, 1, 0) x (1, 0, 0)
  line L0 (-3.6078, -4.9) -> (3.3922, -4.9) projected
  line L1 (3.3922, -4.9) -> (3.3922, -19.9) projected
  line L2 (3.3922, -19.9) -> (-3.6078, -19.9) projected
  line L3 (-3.6078, -19.9) -> (-3.6078, -4.9) projected
  line L4 (6.4642, -4.9) -> (13.4642, -4.9) projected
  line L5 (13.4642, -4.9) -> (13.4642, -19.9) projected
  line L6 (13.4642, -19.9) -> (6.4642, -19.9) projected
  line L7 (6.4642, -19.9) -> (6.4642, -4.9) projected
  line L8 (17.5932, -23.9) -> (17.5932, -11.7729) projected
  line L9 (17.5932, -23.9) -> (17.5932, -22.4)
  line L10 (3.3922, -22.4) -> (-3.6078, -22.4)
  line L11 (-3.6078, -22.4) -> (-3.6078, -4.9)
  line L12 (-3.6078, -4.9) -> (3.3922, -4.9)
  line L13 (3.3922, -4.9) -> (3.3922, -22.4)
  line L14 (13.4642, -22.4) -> (6.4642, -22.4)
  line L15 (6.4642, -22.4) -> (6.4642, -4.9)
  line L16 (6.4642, -4.9) -> (13.4642, -4.9)
  line L17 (13.4642, -4.9) -> (13.4642, -22.4)
  point P0 (0, 0)
  constraints: 18 end point, 4 parallel, 2 horizontal, 2 perpendicular, 1 point on line
extrude "Extrusion64" cut sketch "Sketch69" against normal blind 1.5 contours L2 L13 L10 L11 | L6 L17 L14 L15
sketch "Sketch70" plane through (0, 1.5, 0) normal (0, 1, 0) x (1, 0, 0)
  line L0 (3.3922, -22.4) -> (-3.6078, -22.4) projected
  line L1 (6.4642, -22.4) -> (6.4642, -4.9) projected
  line L2 (6.4642, -4.9) -> (13.4642, -4.9) projected
  line L3 (13.4642, -4.9) -> (13.4642, -22.4) projected
  line L4 (13.4642, -22.4) -> (6.4642, -22.4) projected
  line L5 (-17.5932, -23.9) -> (-17.5932, -11.7729) projected
  line L6 (3.3922, -22.4) -> (3.3922, -22.9)
  line L7 (3.3922, -22.9) -> (-3.6078, -22.9)
  line L8 (-3.6078, -22.9) -> (-3.6078, -22.4)
  line L9 (-3.6078, -22.4) -> (3.3922, -22.4)
  line L10 (3.3922, -22.9) -> (-3.6078, -22.9)
  line L11 (-3.6078, -22.9) -> (-3.6078, -4.9)
  line L12 (-3.6078, -4.9) -> (3.3922, -4.9)
  line L13 (3.3922, -4.9) -> (3.3922, -22.9)
  line L14 (13.4642, -22.9) -> (6.4642, -22.9)
  line L15 (6.4642, -22.9) -> (6.4642, -4.9)
  line L16 (6.4642, -4.9) -> (13.4642, -4.9)
  line L17 (13.4642, -4.9) -> (13.4642, -22.9)
  point P0 (0, 0)
  dimension "d343" = 0.5
  dimension "d344" = 7
  dimension "d345" = 18
  dimension "d346" = 7
  constraints: 24 end point, 6 parallel, 3 perpendicular, 2 horizontal, 1 collinear
  measures "d343" distance of L0.start L6.end
  measures "d344" distance of L11.end L12.end
  measures "d345" distance of L10.end L11.end
  measures "d346" distance of L1.end L16.end